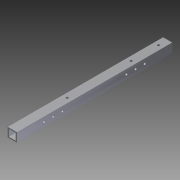
# Autodesk Inventor part: 12 in tube
Saved by Autodesk Inventor 2011 SP1 (Build 150282100, 282)
## iProperties
Created: 2012-01-20
Part Number: 12 in tube
Document SubType Name: Modeling
Designer: Christopher
Density: 1 g/cm^3
Author: Christopher
Autodesk Inventor part; units mm, degrees
ref_plane "YZ Plane" through (0, 0, 0) normal (1, 0, 0) x (0, 1, 0)
ref_plane "XZ Plane" through (0, 0, 0) normal (0, 1, 0) x (-1, 0, 0)
ref_plane "XY Plane" through (0, 0, 0) normal (0, 0, 1) x (1, 0, 0)
sketch "Sketch1" plane through (0, 0, 0) normal (0, 0, 1) x (1, 0, 0)
  line L0 (0, 0) -> (25.4, 0)
  line L1 (25.4, 0) -> (25.4, 25.4)
  line L2 (25.4, 25.4) -> (0, 25.4)
  line L3 (0, 25.4) -> (0, 0)
  line L4 (3.175, 3.175) -> (22.225, 3.175)
  line L5 (22.225, 3.175) -> (22.225, 22.225)
  line L6 (22.225, 22.225) -> (3.175, 22.225)
  line L7 (3.175, 22.225) -> (3.175, 3.175)
  dimension "d0" = 25.4
  dimension "d1" = 25.4
  dimension "d2" = 3.175
  constraints: 16 end point, 4 parallel, 2 perpendicular, 1 horizontal, 3 other
  measures "d0" distance of L1.end L2.end
  measures "d1" distance of L0.end L1.end
  measures "d2" distance between parallel lines of L3 L7
extrude "Extrusion1" add sketch "Sketch1" against normal blind 431.8
sketch "Sketch2" plane through (0, 25.4, 0) normal (0, 1, 0) x (1, 0, 0)
  line L0 (25.4, 431.8) -> (0, 431.8) projected
  point P0 (12.7, 406.4)
  point P1 (12.7, 330.2)
  point P2 (12.7, 152.4)
  dimension "d5" = 25.4
  dimension "d6" = 76.2
  dimension "d7" = 177.8
  measures "d5" distance from line of L0 point (12.7, 406.4)
  measures "d6" distance of point (12.7, 406.4) point (12.7, 330.2)
  measures "d7" distance of point (12.7, 152.4) point (12.7, 330.2)
hole "Hole1" at (12.7, 25.4, -406.4) at (12.7, 25.4, -330.2) at (12.7, 25.4, -152.4) direction (0, -1, 0) diameter 6.35 depth 25.4 tip angle 118
sketch "Sketch3" plane through (25.4, 0, 0) normal (1, 0, 0) x (0, 0, -1)
  line L0 (0, 0) -> (0, 25.4) projected
  line L1 (0, 0) -> (431.8, 0) projected
  line L2 (431.8, 0) -> (431.8, 25.4) projected
  point P0 (63.5, 12.7)
  point P1 (88.9, 12.7)
  point P2 (114.3, 12.7)
  point P3 (342.9, 12.7)
  point P4 (317.5, 12.7)
  point P5 (292.1, 12.7)
  point P6 (431.8, 12.7)
  dimension "d15" = 12.7
  dimension "d16" = 25.4
  dimension "d17" = 25.4
  dimension "d18" = 63.5
  dimension "d26" = 25.4
  dimension "d27" = 25.4
  dimension "d28" = 88.9
  constraints: 5 horizontal alignment, 1 midpoint
  measures "d15" distance from line of L1 point (63.5, 12.7)
  measures "d16" distance of point (88.9, 12.7) point (63.5, 12.7)
  measures "d17" distance of point (114.3, 12.7) point (88.9, 12.7)
  measures "d18" distance from line of L0 point (63.5, 12.7)
  measures "d26" distance of point (317.5, 12.7) point (292.1, 12.7)
  measures "d27" distance of point (342.9, 12.7) point (317.5, 12.7)
  measures "d28" distance from line of L2 point (342.9, 12.7)
hole "Hole2" at (25.4, 12.7, -63.5) at (25.4, 12.7, -88.9) at (25.4, 12.7, -114.3) direction (-1, 0, 0) diameter 6.35 depth 25.4 tip angle 118
hole "Hole3" at (25.4, 12.7, -342.9) at (25.4, 12.7, -317.5) at (25.4, 12.7, -292.1) direction (-1, 0, 0) diameter 6.35 depth 25.4 tip angle 118
body "Solid1"
